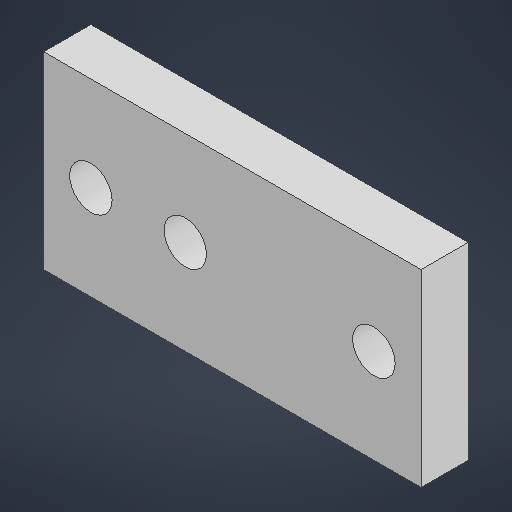
# Autodesk Inventor part: Y Bearing Tensioner
Saved by Autodesk Inventor 2025.1 (Build 291241000, 241)
## iProperties
Created: 2025-03-23
Part Number: Y Bearing Tensioner
Material: Generic
Document SubType Name: Modeling
Designer: jerem
Density: 1 g/cm^3
Appearance: Default
Author: jerem
Autodesk Inventor part; units mm, degrees
ref_plane "YZ Plane" through (0, 0, 0) normal (1, 0, 0) x (0, 1, 0)
ref_plane "XZ Plane" through (0, 0, 0) normal (0, 1, 0) x (-1, 0, 0)
ref_plane "XY Plane" through (0, 0, 0) normal (0, 0, 1) x (1, 0, 0)
sketch "Sketch1" plane through (0, 0, 0) normal (0, 0, 1) x (1, 0, 0)
  circle A0 centre (0, 0) radius 2.25
  circle A1 centre (-10, 0) radius 2.25
  line L0 (-10, 0) -> (0, 0) construction
  line L1 (-15, 10) -> (-15, -10)
  line L2 (-15, -10) -> (25, -10)
  line L3 (-10, 0) -> (-15, 0) construction
  line L4 (-15, 10) -> (25, 10)
  circle A2 centre (20, 0) radius 2.25
  line L5 (20, 0) -> (0, 0) construction
  line L6 (20, 0) -> (25, 0) construction
  line L7 (25, 10) -> (25, -10)
  dimension "d0" = 4.5
  dimension "d1" = 10
  dimension "d2" = 5
  dimension "d3" = 20
  dimension "d4" = 4.5
  dimension "d5" = 20
  dimension "d6" = 5
  constraints: 16 end point, 4 horizontal, 3 centre point, 2 midpoint, 2 vertical, 1 coincident, 1 equal radius, 1 parallel, 1 perpendicular, 1 point on line
  measures "d0" diameter of A1
  measures "d1" distance of L0.start L0.end
  measures "d2" distance of L3.end L0.start
  measures "d3" distance of L1.start L1.end
  measures "d4" diameter of A2
  measures "d5" distance of L5.start L0.end
  measures "d6" distance of L6.end L5.start
extrude "Extrusion1" add sketch "Sketch1" along normal blind 5
body "Solid1"
